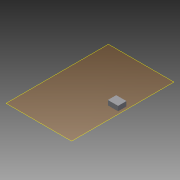
# Autodesk Inventor part: nanopc_t4_headphone
Saved by Autodesk Inventor 2013 SP2 (Build 170200200, 200)
## iProperties
Created: 2018-09-03
Part Number: nanopc_t4_headphone
Material: Generic
Document SubType Name: Modeling
Designer: alex
Density: 1 g/cm^3
Author: alex
Autodesk Inventor part; units mm, degrees
ref_plane "YZ Plane" through (0, 0, 0) normal (1, 0, 0) x (0, 1, 0)
ref_plane "XZ Plane" through (0, 0, 0) normal (0, 1, 0) x (-1, 0, 0)
ref_plane "XY Plane" through (0, 0, 0) normal (0, 0, 1) x (1, 0, 0)
ref_plane "Work Plane1" through (0, 0, 0) normal (0, 0, 1) x (1, 0, 0)
sketch "Sketch1" plane through (0, 0, 0) normal (0, 0, 1) x (1, 0, 0)
  line L0 (21.3787, 6.8051) -> (32.3787, 6.8051)
  line L1 (32.3787, 6.8051) -> (32.3787, -2.1949)
  line L2 (32.3787, -2.1949) -> (21.3787, -2.1949)
  line L3 (21.3787, -2.1949) -> (21.3787, 6.8051)
  point P0 (0, 0)
  dimension "d0" = 11
  dimension "d2" = 9
  constraints: 8 end point, 2 parallel, 1 horizontal, 1 perpendicular
  measures "d0" distance of L1.end L2.end
  measures "d2" distance of L0.end L1.end
extrude "Extrusion1" add sketch "Sketch1" along normal blind 5
sketch "Sketch2" plane through (32.3787, -2.1949, 0) normal (1, 0, 0) x (0, 0, -1)
  circle A0 centre (-2.5, 4.5) radius 3.1
  point P0 (0, 2.1949)
  dimension "d5" = 6.2
  constraints: 1 centre point
  measures "d5" diameter of A0
extrude "Extrusion2" add sketch "Sketch2" along normal blind 4
sketch "Sketch3" plane through (36.3787, 2.3051, 2.5) normal (1, 0, 0) x (0, 0, -1)
  circle A0 centre (0, 0) radius 3.1 projected
  circle A1 centre (0, 0) radius 1.75
  point P0 (2.5, -2.3051)
  dimension "d9" = 3.5
  constraints: 1 centre point, 1 coincident
  measures "d9" diameter of A1
extrude "Extrusion3" cut sketch "Sketch3" against normal blind 7 contours A1
body "Solid1"
